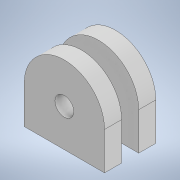
# Autodesk Inventor part: Soporte
Saved by Autodesk Inventor 2021 (Build 250183000, 183)
## iProperties
Created: 2022-01-12
Part Number: Soporte
Material: Generic
Document SubType Name: Modeling
Designer: Yeison
Density: 1 g/cm^3
Appearance: Default
Author: Yeison
Autodesk Inventor part; units mm, degrees
ref_plane "YZ Plane" through (0, 0, 0) normal (1, 0, 0) x (0, 1, 0)
ref_plane "XZ Plane" through (0, 0, 0) normal (0, 1, 0) x (-1, 0, 0)
ref_plane "XY Plane" through (0, 0, 0) normal (0, 0, 1) x (1, 0, 0)
sketch "Sketch1" plane through (0, 0, 0) normal (0, 0, 1) x (1, 0, 0)
  circle A0 centre (0, 0) radius 5.5
  line L0 (5.5, 0) -> (23.5, 0)
  line L1 (-5.5, 0) -> (-23.5, 0)
  arc A1 (23.5, 0) -> (-23.5, 0) centre (0, 0) ccw
  line L2 (-23.5, 0) -> (-23.5, -22)
  line L3 (-23.5, 0) -> (-1.5, 0) construction
  line L4 (-23.5, -22) -> (23.5, -22)
  line L5 (23.5, -22) -> (23.5, 0)
  dimension "d0" = 11
  dimension "d1" = 18
  dimension "d2" = 18
  dimension "d3" = 22
  dimension "d4" = 90
  constraints: 12 end point, 4 point on circle, 3 horizontal, 3 perpendicular, 2 centre point, 2 coincident, 1 point on line, 1 vertical
  measures "d0" diameter of A0
  measures "d1" distance of L0.start L0.end
  measures "d2" distance of L1.start L1.end
  measures "d3" distance of L2.start L2.end
  measures "d4" angle of L2 L3
extrude "Extrusion1" add sketch "Sketch1" against normal blind 10 contours L0 L5 L4 L2 L1 A0 | A0 L1 A1 L0
ref_plane "Work Plane1" through (0, 0, -15) normal (0, 0, -1) x (1, 0, 0)
mirror "Mirror1" about plane through (0, 0, -15) normal (0, 0, -1) of "Extrusion1"
ref_plane "Work Plane2" through (-23.5, -22, -10) normal (0, -1, 0) x (-1, 0, 0)
body "Solid1"
